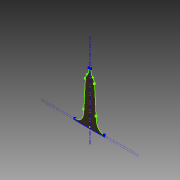
# Autodesk Inventor part: Bottom Plate
Saved by Autodesk Inventor 2012 (Build 160160000, 160)
## iProperties
Created: 2013-02-28
Part Number: Bottom Plate
Material: Wood (Cherry)
Document SubType Name: Modeling
Designer: fixer
Mass: 55.5644 g
Surface Area: 736.311 cm^2
Volume: 111.129 cm^3
Density: 0.5 g/cm^3
Author: fixer
Autodesk Inventor part; units mm, degrees
ref_plane "YZ Plane" through (0, 0, 0) normal (1, 0, 0) x (0, 1, 0)
ref_plane "XZ Plane" through (0, 0, 0) normal (0, 1, 0) x (-1, 0, 0)
ref_plane "XY Plane" through (0, 0, 0) normal (0, 0, 1) x (1, 0, 0)
sketch "Sketch1" plane through (0, 0, 0) normal (0, 0, 1) x (1, 0, 0)
  line L0 (76.2, -12.7) -> (381, -12.7) construction
  line L1 (-76.2, -12.7) -> (-381, -12.7) construction
  line L2 (-76.2, 0) -> (-381, 0) construction
  line L3 (76.2, 0) -> (381, 0) construction
  line L4 (0, -116.2267) -> (0, 608.4603)
  line L5 (0, -12.7) -> (-114.3, -12.7)
  line L6 (-114.3, -12.7) -> (-114.3, 0)
  line L7 (0, 393.7) -> (-6.35, 393.7)
  line L8 (-35.6495, 307.6636) -> (-47.1726, 94.4804)
  spline S0 degree 3 poles (-114.3, 0) (-54.5856, 0) (-49.4191, 52.9191) (-47.1726, 94.4804) knots 0 0 0 0 1 1 1 1
  line L9 (-119.6474, 0) -> (-108.9526, 0) construction
  arc A0 (-118.5741, 0.0908) -> (-110.0259, 0.0904) centre (-114.3, 101.0734) ccw construction
  line L10 (35.6495, 307.6636) -> (47.1726, 94.4804)
  line L11 (0, 393.7) -> (6.35, 393.7)
  spline S1 degree 3 poles (114.3, 0) (54.5856, 0) (49.4191, 52.9191) (47.1726, 94.4804) knots 0 0 0 0 1 1 1 1
  line L12 (119.6474, 0) -> (108.9526, 0) construction
  arc A1 (110.0259, 0.0904) -> (118.5741, 0.0908) centre (114.3, 101.0734) ccw construction
  line L13 (0, -12.7) -> (114.3, -12.7)
  line L14 (114.3, -12.7) -> (114.3, 0)
  spline S2 degree 4 poles (-6.35, 393.7) (-6.35, 372.311) (-15.6243, 344.3546) (-23.8914, 342.6208) (-35.1144, 317.5619) (-35.6495, 307.6636) knots 0 0 0 0 0 0.524924 1 1 1 1 1
  line L15 (-6.35, 420.5818) -> (-6.35, 366.8182) construction
  arc A2 (-8.1557, 372.5045) -> (-8.1557, 414.8955) centre (-131.6479, 393.7) ccw construction
  spline S3 degree 4 poles (6.35, 393.7) (6.35, 352.9531) (17.6853, 348.1201) (34.5233, 328.4987) (35.6495, 307.6636) knots 0 0 0 0 0 1 1 1 1 1
  line L16 (6.35, 420.5818) -> (6.35, 366.8182) construction
  arc A3 (8.1557, 414.8955) -> (8.1557, 372.5045) centre (131.6479, 393.7) ccw construction
  line L17 (-14.8603, 351.5845) -> (-28.3954, 331.1958) construction
  arc A4 (-16.1968, 349.5342) -> (-27.0248, 333.2235) centre (1931.9258, -955.4859) ccw construction
  point P0 (0, 0)
  point P1 (-21.6278, 341.3901)
  point P2 (21.6278, 341.3901)
  dimension "d0" = 6.35
  dimension "d3" = 114.3
  dimension "d4" = 406.4
  constraints: 36 end point, 16 symmetric about line, 9 horizontal, 8 midpoint, 5 point on line, 5 vertical, 3 centre point, 3 point on circle, 2 perpendicular, 26 other
  measures "d0" distance of L7.start L7.end
  measures "d3" distance of L5.start L13.end
  measures "d4" distance between parallel lines of L13 L11
extrude "Extrusion1" add sketch "Sketch1" against normal blind 3.175
body "Solid1"
